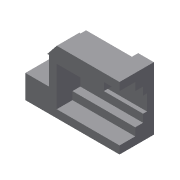
# Autodesk Inventor part: connect
Saved by Autodesk Inventor 2022 (Build 260148000, 148)
## iProperties
Shininess: 64.0
Length Units: 11269
Angle Units: 11279
Time Units: 11290
Mass Units: 11283
Length Display Precision: 3
Angle Display Precision: 2
Created: 2002-02-13
Part Number: connect
Document SubType Name: Modeling
Designer: Administrator
Density: 1 g/cm^3
Material: Generic
Appearance: Default
Density: 0.0
Volumn: 0.0
Area: 0.0
PropertySet Name: Model Information
Control State: 0
Master: False
Checked Out: False
Author: Administrator
Autodesk Inventor part; units mm, degrees
ref_plane "YZ Plane" through (0, 0, 0) normal (1, 0, 0) x (0, 1, 0)
ref_plane "XZ Plane" through (0, 0, 0) normal (0, 1, 0) x (-1, 0, 0)
ref_plane "XY Plane" through (0, 0, 0) normal (0, 0, 1) x (1, 0, 0)
sketch "Sketch1" plane through (0, 0, 0) normal (0, 0, 1) x (1, 0, 0)
  line L0 (-11.4074, 18.7393) -> (-11.4074, 6.0393)
  line L1 (-11.4074, 6.0393) -> (-30.4574, 6.0393)
  line L2 (-30.4574, 6.0393) -> (-30.4574, 10.8018)
  line L3 (-30.4574, 10.8018) -> (-24.1074, 18.7393)
  line L4 (-11.4074, 18.7393) -> (-24.1074, 18.7393)
  dimension "d0" = 12.7
  dimension "d1" = 19.05
  dimension "d2" = 4.7625
  dimension "d4" = 12.7
  constraints: 11 end point, 2 perpendicular, 1 parallel, 1 vertical
  measures "d0" distance of L0.start L0.end
  measures "d1" distance of L0.end L1.end
  measures "d2" distance of L1.end L2.end
  measures "d4" distance of L0.start L3.end
extrude "Extrusion1" add sketch "Sketch1" along normal blind 13.8906
sketch "Sketch3" plane through (-30.4574, 6.0393, 0) normal (-1, 0, 0) x (0, 0, 1)
  line L0 (13.8906, 0) -> (13.8906, 4.7625) projected
  line L1 (0, 4.7625) -> (13.8906, 4.7625) projected
  line L2 (0, 0) -> (0, 4.7625) projected
  line L3 (0, 0) -> (13.8906, 0) projected
  circle A0 centre (6.9453, 2.1164) radius 6.9453 construction
  line L4 (6.9453, 2.1164) -> (6.9453, 0)
  constraints: 2 end point, 2 tangent, 1 centre point, 1 midpoint, 1 perpendicular
ref_plane "Work Plane1" through (-30.4574, 8.1557, 6.9453) normal (0, 0, -1) x (-1, 0, 0)
sketch "Sketch4" plane through (-30.4574, 8.1557, 6.9453) normal (0, 0, -1) x (-1, 0, 0)
  line L0 (-4.7625, 8.2023) -> (0, 8.2023)
  line L1 (0, 8.2023) -> (0, 2.6461)
  line L2 (0, 2.6461) -> (-4.7625, 2.6461)
  line L3 (-4.7625, 2.6461) -> (-4.7625, 8.2023)
  line L4 (0, -2.1164) -> (0, 2.6461) projected
  dimension "d13" = 4.7625
  dimension "d14" = 5.5563
  constraints: 8 end point, 2 parallel, 1 collinear, 1 horizontal, 1 perpendicular
  measures "d13" distance of L1.end L2.end
  measures "d14" distance of L0.end L1.end
extrude "Extrusion3" cut sketch "Sketch4" against normal mid plane 9.525
sketch "Sketch5" plane through (-11.4074, 6.0393, 0) normal (1, 0, 0) x (0, 0, -1)
  line L0 (-13.8906, 12.7) -> (-13.8906, 0) projected
  line L1 (0, 0) -> (-13.8906, 0) projected
  line L2 (0, 12.7) -> (0, 0) projected
  line L3 (0, 12.7) -> (-13.8906, 12.7) projected
  line L4 (-11.7078, 9.525) -> (-2.1828, 9.525)
  line L5 (-2.1828, 9.525) -> (-2.1828, 3.175)
  line L6 (-2.1828, 3.175) -> (-11.7078, 3.175)
  line L7 (-11.7078, 3.175) -> (-11.7078, 9.525)
  circle A0 centre (-6.9453, 6.35) radius 4.7625 construction
  circle A1 centre (-6.9453, 6.35) radius 3.175 construction
  circle A2 centre (-6.9453, 6.35) radius 6.35 construction
  circle A3 centre (-6.9453, 6.35) radius 6.9453 construction
  dimension "d17" = 9.525
  dimension "d18" = 6.35
  constraints: 8 end point, 8 tangent, 4 centre point, 3 coincident, 2 parallel, 1 horizontal, 1 perpendicular
  measures "d17" distance of L5.end L6.end
  measures "d18" distance of L4.end L5.end
extrude "Extrusion4" cut sketch "Sketch5" against normal blind 12.7 contours L4 L5 L6 L7
sketch "Sketch6" plane through (-11.4074, 6.0393, 0) normal (1, 0, 0) x (0, 0, -1)
  line L0 (-11.7078, 3.175) -> (-11.7078, 9.525) projected
  line L1 (-11.7078, 9.525) -> (-2.1828, 9.525) projected
  line L2 (-2.1828, 9.525) -> (-2.1828, 3.175) projected
  line L3 (-10.1203, 9.525) -> (-3.7703, 9.525)
  line L4 (-3.7703, 9.525) -> (-3.7703, 11.1125)
  line L5 (-3.7703, 11.1125) -> (-10.1203, 11.1125)
  line L6 (-10.1203, 11.1125) -> (-10.1203, 9.525)
  circle A0 centre (-6.9453, 20.5431) radius 3.175 construction
  circle A1 centre (-6.9453, 20.5431) radius 4.7625 construction
  dimension "d21" = 6.35
  dimension "d22" = 1.5875
  constraints: 8 end point, 4 tangent, 2 centre point, 2 parallel, 1 collinear, 1 concentric, 1 horizontal, 1 perpendicular
  measures "d21" distance of L4.end L5.end
  measures "d22" distance of L3.end L4.end
extrude "Extrusion5" cut sketch "Sketch6" against normal blind 3.175
sketch "Sketch7" plane through (-11.4074, 6.0393, 0) normal (1, 0, 0) x (0, 0, -1)
  line L0 (-13.8906, 12.7) -> (-13.8906, 0) projected
  line L1 (0, 0) -> (-13.8906, 0) projected
  line L2 (0, 12.7) -> (0, 0) projected
  line L3 (0, 12.7) -> (-13.8906, 12.7) projected
  line L4 (-12.5016, 7.9375) -> (-1.3891, 7.9375)
  line L5 (-1.3891, 7.9375) -> (-1.3891, 4.7625)
  line L6 (-1.3891, 4.7625) -> (-12.5016, 4.7625)
  line L7 (-12.5016, 4.7625) -> (-12.5016, 7.9375)
  circle A0 centre (-6.9453, 6.35) radius 5.5563 construction
  circle A1 centre (-6.9453, 6.35) radius 6.9453 construction
  circle A2 centre (-6.9453, 6.35) radius 6.35 construction
  circle A3 centre (-6.9453, 6.35) radius 1.5875 construction
  dimension "d25" = 3.175
  dimension "d26" = 11.1125
  constraints: 8 end point, 8 tangent, 4 centre point, 3 concentric, 2 parallel, 1 horizontal, 1 perpendicular
  measures "d25" distance of L6.end L4.start
  measures "d26" distance of L4.start L4.end
extrude "Extrusion6" cut sketch "Sketch7" against normal blind 9.525 contours L4 L5 L6 L7
sketch "Sketch8" plane through (-11.4074, 6.0393, 0) normal (1, 0, 0) x (0, 0, -1)
  line L0 (-10.1203, 9.525) -> (-10.1203, 11.1125) projected
  line L1 (-3.7703, 11.1125) -> (-3.7703, 9.525) projected
  line L2 (-2.1828, 3.175) -> (-11.7078, 3.175) projected
  line L3 (-10.1203, 3.175) -> (-3.7703, 3.175)
  line L4 (-3.7703, 3.175) -> (-3.7703, 1.5875)
  line L5 (-3.7703, 1.5875) -> (-10.1203, 1.5875)
  line L6 (-10.1203, 1.5875) -> (-10.1203, 3.175)
  dimension "d29" = 1.5875
  constraints: 8 end point, 3 collinear, 2 parallel, 1 horizontal, 1 perpendicular
  measures "d29" distance of L5.end L3.start
extrude "Extrusion7" cut sketch "Sketch8" against normal up to surface (12.7 mm away)
sketch "Sketch9" plane through (-30.4574, 6.0393, 0) normal (0, -1, 0) x (1, 0, 0)
  line L0 (19.05, 13.8906) -> (0, 13.8906) projected
  line L1 (19.05, 0) -> (0, 0) projected
  line L2 (19.05, 0) -> (19.05, 13.8906) projected
  line L3 (11.5094, -0.1544) -> (11.5094, 2.9198)
  line L4 (11.5094, 10.9708) -> (11.5094, 14.045)
  line L5 (10.7156, -0.1544) -> (10.7156, 2.9198)
  line L6 (10.7156, 10.9708) -> (10.7156, 14.045)
  arc A0 (10.7156, 2.9198) -> (10.7156, -0.1544) centre (11.1125, 1.3827) ccw
  arc A1 (11.5094, -0.1544) -> (11.5094, 2.9198) centre (11.1125, 1.3827) ccw
  arc A2 (11.5094, 10.9708) -> (11.5094, 14.045) centre (11.1125, 12.5079) ccw
  arc A3 (10.7156, 14.045) -> (10.7156, 10.9708) centre (11.1125, 12.5079) ccw
  circle A4 centre (11.1125, 6.9453) radius 5.5626 construction
  circle A5 centre (11.1125, 6.9453) radius 6.9453 construction
  dimension "d32" = 7.9375
  dimension "d33" = 1.5875
  dimension "d34" = 0.7937
  dimension "d35" = 0.3969
  dimension "d45" = 11.1252
  constraints: 10 point on circle, 8 end point, 6 centre point, 4 parallel, 3 equal radius, 2 collinear, 2 tangent, 1 concentric, 1 vertical, 1 vertical alignment
  measures "d32" distance from line of L2 A0.centre
  measures "d33" radius of A3
  measures "d34" distance of L3.end L5.end
  measures "d35" distance from line of A0.centre L5
  measures "d45" distance of A0.centre A2.centre
extrude "Extrusion8" add sketch "Sketch9" along normal blind 3.175
sketch "Sketch10" plane through (-24.1074, 18.7393, 0) normal (0, 1, 0) x (1, 0, 0)
  line L0 (0, -13.8906) -> (12.7, -13.8906) projected
  line L1 (12.7, 0) -> (12.7, -13.8906) projected
  line L2 (0, 0) -> (12.7, 0) projected
  line L3 (9.525, 0) -> (-3.175, 0)
  line L4 (-3.175, 0) -> (-3.175, -2.3813)
  line L5 (-3.175, -2.3813) -> (9.525, -2.3812)
  line L6 (9.525, -2.3812) -> (9.525, 0)
  line L7 (9.525, -11.5094) -> (-3.175, -11.5094)
  line L8 (-3.175, -11.5094) -> (-3.175, -13.8906)
  line L9 (-3.175, -13.8906) -> (9.525, -13.8906)
  line L10 (9.525, -13.8906) -> (9.525, -11.5094)
  dimension "d38" = 3.175
  dimension "d39" = 2.3813
  dimension "d40" = 2.3813
  dimension "d41" = 12.7
  dimension "d42" = 12.7
  constraints: 16 end point, 4 parallel, 2 collinear, 2 horizontal, 2 perpendicular, 1 point on line
  measures "d38" distance between parallel lines of L1 L6
  measures "d39" distance of L5.end L3.start
  measures "d40" distance of L9.end L7.start
  measures "d41" distance of L9.end L8.end
  measures "d42" distance of L4.end L5.end
extrude "Extrusion9" cut sketch "Sketch10" against normal blind 1.27
ref_plane "Work Plane2" through (0, 0, 6.9453) normal (0, 0, 1) x (1, 0, 0)
sketch "Sketch12" plane through (0, 0, 6.9453) normal (0, 0, 1) x (1, 0, 0)
  line L0 (-34.925, 19.05) -> (-7.9375, 19.05)
  line L1 (-7.9375, 19.05) -> (-7.9375, -1.5875)
  line L2 (-7.9375, -1.5875) -> (-34.925, -1.5875)
  line L3 (-34.925, -1.5875) -> (-34.925, 19.05)
  constraints: 8 end point, 2 parallel, 1 horizontal, 1 perpendicular
extrude "Extrusion10" cut sketch "Sketch12" along normal through all
body "Solid1"
